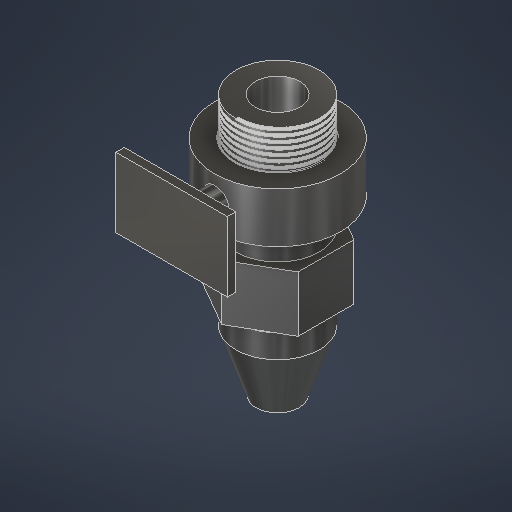
# Autodesk Inventor part: Part2
Saved by Autodesk Inventor 2026 (Build 300175000, 175)
## iProperties
Created: 2023-09-18
Part Number: Part2
Material: Generic
Document SubType Name: Modeling
Designer: gzb
Density: 1 g/cm^3
Appearance: Default
Author: gzb
Autodesk Inventor part; units mm, degrees
ref_plane "YZ Plane" through (0, 0, 0) normal (1, 0, 0) x (0, 1, 0)
ref_plane "XZ Plane" through (0, 0, 0) normal (0, 1, 0) x (-1, 0, 0)
sketch "Sketch1" plane through (0, 0, 0) normal (0, 0, 1) x (1, 0, 0)
  line L0 (0, 0) -> (0, 93.5)
  line L1 (0, 93.5) -> (15, 93.5)
  line L2 (15, 93.5) -> (15, 80)
  line L3 (15, 80) -> (22.5, 80)
  line L4 (22.5, 80) -> (22.5, 62)
  line L5 (22.5, 62) -> (15, 62)
  line L6 (15, 62) -> (15, 21.6)
  line L7 (15, 21.6) -> (7.75, 0)
  line L8 (7.75, 0) -> (0, 0)
  dimension "d0" = 93.5
  dimension "d1" = 18
  dimension "d2" = 58.4
  dimension "d3" = 80
  dimension "d4" = 45
  dimension "d5" = 30
  dimension "d6" = 15.5
  constraints: 18 end point, 5 perpendicular, 2 point on line, 1 parallel, 1 vertical
  measures "d0" distance of L0.start L0.end
  measures "d1" distance of L3.end L4.end
  measures "d2" distance from line of L6.end L3
  measures "d3" distance between parallel lines of L3 L8
  measures "d4" diameter of L4 L0
  measures "d5" diameter of L6 L0
  measures "d6" diameter of L7.end L0
revolve "Revolution1" add sketch "Sketch1" angle 360 about axis through (0, 0, 0) along (0, 1, 0)
ref_plane "Work Plane1" through (0, 52, 0) normal (0, 1, 0) x (1, 0, 0)
sketch "Sketch2" plane through (0, 52, 0) normal (0, 1, 0) x (1, 0, 0)
  line L0 (0, 20.0629) -> (17.375, 10.0315)
  line L1 (17.375, 10.0315) -> (17.375, -10.0315)
  line L2 (17.375, -10.0315) -> (0, -20.0629)
  line L3 (0, -20.0629) -> (-17.375, -10.0315)
  line L4 (-17.375, -10.0315) -> (-17.375, 10.0315)
  line L5 (-17.375, 10.0315) -> (0, 20.0629)
  point P0 (0, 0)
  point P1 (0, 0)
  dimension "d9" = 34.75
  constraints: 12 end point, 1 coincident, 1 vertical alignment, 13 other
  measures "d9" distance between parallel lines of L1 L4
extrude "Extrusion1" add sketch "Sketch2" against normal blind 20
sketch "Sketch4" plane through (0, 0, 0) normal (1, 0, 0) x (0, 1, 0)
  line L0 (93.5, 15) -> (93.5, -15) projected
  line L1 (93.5, 0) -> (0, 0)
  line L2 (93.5, 0) -> (93.5, 8)
  line L3 (93.5, 8) -> (68.5, 8)
  line L4 (68.5, 8) -> (68.5, 13)
  line L5 (68.5, 13) -> (52.5, 13)
  line L6 (52.5, 13) -> (52.5, 2.85)
  line L7 (52.5, 2.85) -> (50.5, 2.85)
  line L8 (50.5, 2.85) -> (50.5, 8)
  line L9 (50.5, 8) -> (20.5, 8)
  line L10 (20.5, 8) -> (20.5, 4.75)
  line L11 (20.5, 4.75) -> (3, 4.75)
  line L12 (3, 4.75) -> (0, 1.75)
  line L13 (0, 1.75) -> (0, 0)
  line L14 (0, 7.75) -> (0, -7.75) projected
  dimension "d21" = 25
  dimension "d22" = 16
  dimension "d23" = 2
  dimension "d24" = 30
  dimension "d25" = 17.5
  dimension "d26" = 45
  dimension "d27" = 16
  dimension "d28" = 26
  dimension "d29" = 5.7
  dimension "d30" = 16
  dimension "d31" = 9.5
  constraints: 26 end point, 8 perpendicular, 2 horizontal, 1 collinear, 1 midpoint, 1 point on line
  measures "d21" distance of L2.end L3.end
  measures "d22" distance of L4.end L5.end
  measures "d23" distance between parallel lines of L8 L6
  measures "d24" distance of L8.end L9.end
  measures "d25" distance from line of L11.end L10
  measures "d26" angle of L12 L14
  measures "d27" diameter of L3 L1
  measures "d28" diameter of L5 L1
  measures "d29" diameter of L7 L1
  measures "d30" diameter of L9 L1
  measures "d31" diameter of L11 L1
revolve "Revolution2" cut sketch "Sketch4" angle 360 about axis through (0, 93.5, 0) along (0, -1, 0)
ref_plane "Work Plane2" through (0, 0, 35) normal (0, 0, 1) x (1, 0, 0)
sketch "Sketch6" plane through (0, 0, 35) normal (0, 0, 1) x (1, 0, 0)
  circle A0 centre (0, 72) radius 4.375
  line L0 (-22.5, 80) -> (22.5, 80) projected
  point P0 (0, 0)
  dimension "d35" = 8.75
  dimension "d36" = 8
  constraints: 1 centre point, 1 vertical alignment
  measures "d35" diameter of A0
  measures "d36" distance from line of A0.centre L0
extrude "Extrusion2" add sketch "Sketch6" against normal up to next
sketch "Sketch7" plane through (0, 72, 35) normal (0, 0, 1) x (1, 0, 0)
  circle A0 centre (0, 0) radius 4.375 projected
  circle A1 centre (0, 0) radius 3
  point P0 (0, -72)
  dimension "d39" = 6
  constraints: 1 centre point, 1 coincident
  measures "d39" diameter of A1
extrude "Extrusion3" cut sketch "Sketch7" against normal blind 34.75 contours A1
chamfer "Chamfer1" distance 3 angle 45 1 edges at (-15, 62, 0)
chamfer "Chamfer2" distance 2 angle 45 1 edges at (-15, 32, 0)
sketch "Sketch8" plane through (0, 93.5, 0) normal (0, 1, 0) x (1, 0, 0)
  circle A0 centre (0, 0) radius 15 projected
ref_plane "Work Plane3" through (0, 93.5, 15) normal (0.9997749, -0.0212159, 0) x (0.0212159, 0.9997749, 0)
sketch "Sketch9" plane through (0, 93.5, 15) normal (0.9997749, -0.0212159, 0) x (0.0212159, 0.9997749, 0)
  line L0 (0, -0.866) -> (-0.75, 0.433)
  line L1 (-0.75, 0.433) -> (0.75, 0.433)
  line L2 (0.75, 0.433) -> (0, -0.866)
  point P0 (-93.479, -15)
  point P1 (0, 0)
  point P2 (0, 0)
  point P3 (0, 0.433)
  dimension "d60" = 1.5
  constraints: 6 end point, 1 coincident, 1 midpoint, 1 vertical alignment, 7 other
  measures "d60" distance of L0.end L1.end
sketch3d "3D Sketch3"
  helix H0 starts at (0, 93.5, 15) axis through (0, 93.5, 0) along (0, -1, 0) pitch 2 turns 12 hand left
sweep "Sweep1" cut profiles "Sketch9" path "3D Sketch3"
sketch "Sketch10" plane through (0, 72, 35) normal (0, 0, 1) x (1, 0, 0)
  line L0 (-20, 12.5) -> (20, 12.5)
  line L1 (20, 12.5) -> (20, -12.5)
  line L2 (20, -12.5) -> (-20, -12.5)
  line L3 (-20, -12.5) -> (-20, 12.5)
  circle A0 centre (0, 0) radius 4.375 projected
  point P0 (0, -72)
  point P1 (-20, 0)
  point P2 (0, -12.5)
  dimension "d63" = 25
  dimension "d64" = 40
  constraints: 8 end point, 2 midpoint, 2 parallel, 1 horizontal, 1 horizontal alignment, 1 perpendicular, 1 vertical alignment
  measures "d63" distance of L0.end L1.end
  measures "d64" distance of L1.end L2.end
extrude "Extrusion4" add sketch "Sketch10" along normal blind 3 contours L0 L1 L2 L3 | A0
body "Solid1"
